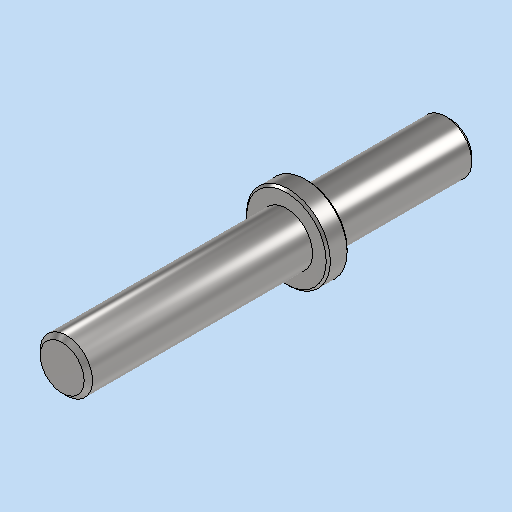
# Autodesk Inventor part: rail-shaft
Saved by Autodesk Inventor 2025 (Build 290162000, 162)
## iProperties
Created: 2025-05-28
Part Number: rail-shaft
Material: Stainless Steel
Document SubType Name: Modeling
Designer: kuzmin
Density: 8 g/cm^3
Appearance: Semi-Polished
Author: kuzmin
Autodesk Inventor part; units mm, degrees
ref_plane "YZ Plane" through (0, 0, 0) normal (1, 0, 0) x (0, 1, 0)
ref_plane "XZ Plane" through (0, 0, 0) normal (0, 1, 0) x (-1, 0, 0)
ref_plane "XY Plane" through (0, 0, 0) normal (0, 0, 1) x (1, 0, 0)
sketch "Sketch1" plane through (0, 0, 0) normal (1, 0, 0) x (0, 1, 0)
  line L0 (0, -13.6) -> (0, 23.4)
  line L1 (0, 23.4) -> (2.5, 23.4)
  line L2 (2.5, 23.4) -> (2.5, 2)
  line L3 (2.5, 2) -> (4, 2)
  line L4 (4, 2) -> (4, 0)
  line L5 (4, 0) -> (2.5, 0)
  line L6 (2.5, 0) -> (2.5, -13.6)
  line L7 (2.5, -13.6) -> (0, -13.6)
  point P0 (0, 0)
  dimension "d0" = 5
  dimension "d1" = 37
  dimension "d2" = 13.6
  dimension "d3" = 2
  dimension "d4" = 8
  constraints: 16 end point, 6 perpendicular, 3 point on line, 1 horizontal alignment, 1 vertical
  measures "d0" diameter of L2 L0
  measures "d1" distance of L0.start L0.end
  measures "d2" distance of L5.end L6.end
  measures "d3" distance of L3.end L4.end
  measures "d4" diameter of L4 L0
revolve "Revolution1" add sketch "Sketch1" angle 360 about axis through (0, 0, -13.6) along (0, 0, 1)
chamfer "Chamfer1" distance 0.4 angle 45 2 edges at (0, -2.5, -13.6) (0, -2.5, 23.4)
chamfer "Chamfer2" distance 0.2 angle 45 2 edges at (0, -4, 2) (0, -4, 0)
body "Solid1"
